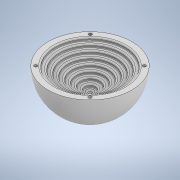
# Autodesk Inventor part: Energy_D
Saved by Autodesk Inventor 2022 (Build 260153000, 153)
## iProperties
Created: 2021-10-08
Part Number: Energy_D
Material: 一般
Document SubType Name: Modeling
Designer: zz091
Density: 1 g/cm^3
Appearance: 預設
Author: zz091
Autodesk Inventor part; units mm, degrees
ref_plane "YZ Plane" through (0, 0, 0) normal (1, 0, 0) x (0, 1, 0)
ref_plane "XZ Plane" through (0, 0, 0) normal (0, 1, 0) x (-1, 0, 0)
ref_plane "XY Plane" through (0, 0, 0) normal (0, 0, 1) x (1, 0, 0)
sketch "草圖3" plane through (0, 0, 0) normal (0, 1, 0) x (-1, 0, 0)
  circle A0 centre (0, 0) radius 30
  dimension "d1" = 60
  constraints: 1 centre point, 1 coincident
  measures "d1" diameter of A0
extrude "擠出1" add sketch "草圖3" against normal blind 30
fillet "圓角1" radius 30 1 edges at (30, -30, 0)
sketch "草圖4" plane through (0, 0, 0) normal (0, 1, 0) x (1, 0, 0)
  circle A0 centre (0, 0) radius 25
  dimension "d6" = 50
  constraints: 1 centre point, 1 coincident
  measures "d6" diameter of A0
extrude "擠出2" cut sketch "草圖4" against normal blind 2
sketch "草圖5" plane through (0, -2, 0) normal (0, 1, 0) x (1, 0, 0)
  circle A0 centre (0, 0) radius 22
  dimension "d9" = 44
  constraints: 1 centre point, 1 coincident
  measures "d9" diameter of A0
extrude "擠出3" cut sketch "草圖5" against normal blind 2
sketch "草圖6" plane through (0, -4, 0) normal (0, 1, 0) x (1, 0, 0)
  circle A0 centre (0, 0) radius 19
  dimension "d12" = 38
  constraints: 1 centre point, 1 coincident
  measures "d12" diameter of A0
extrude "擠出4" cut sketch "草圖6" against normal blind 2
sketch "草圖7" plane through (0, -6, 0) normal (0, 1, 0) x (1, 0, 0)
  circle A0 centre (0, 0) radius 16
  dimension "d15" = 32
  constraints: 1 centre point, 1 coincident
  measures "d15" diameter of A0
extrude "擠出5" cut sketch "草圖7" against normal blind 2
sketch "草圖8" plane through (0, -8, 0) normal (0, 1, 0) x (1, 0, 0)
  circle A0 centre (0, 0) radius 13
  dimension "d18" = 26
  constraints: 1 centre point, 1 coincident
  measures "d18" diameter of A0
extrude "擠出6" cut sketch "草圖8" against normal blind 2
sketch "草圖9" plane through (0, -10, 0) normal (0, 1, 0) x (1, 0, 0)
  circle A0 centre (0, 0) radius 10
  dimension "d21" = 20
  constraints: 1 centre point, 1 coincident
  measures "d21" diameter of A0
extrude "擠出7" cut sketch "草圖9" against normal blind 2
sketch "草圖10" plane through (0, -12, 0) normal (0, 1, 0) x (1, 0, 0)
  circle A0 centre (0, 0) radius 7
  dimension "d24" = 14
  constraints: 1 centre point, 1 coincident
  measures "d24" diameter of A0
extrude "擠出8" cut sketch "草圖10" against normal blind 2
sketch "草圖11" plane through (0, -14, 0) normal (0, 1, 0) x (1, 0, 0)
  circle A0 centre (0, 0) radius 4
  dimension "d27" = 8
  constraints: 1 centre point, 1 coincident
  measures "d27" diameter of A0
extrude "擠出9" cut sketch "草圖11" against normal blind 2
sketch "草圖14" plane through (0, -16, 0) normal (0, 1, 0) x (1, 0, 0)
  circle A0 centre (0, 0) radius 7 projected
  circle A1 centre (0, 0) radius 1.5
  dimension "d33" = 3
  constraints: 1 centre point, 1 coincident
  measures "d33" diameter of A1
extrude "擠出11" cut sketch "草圖14" against normal blind 2 contours A1
sketch "草圖15" plane through (0, 0, 0) normal (1, 0, 0) x (0, 1, 0)
  circle A0 centre (0, 0) radius 1.5
  dimension "d36" = 3
  constraints: 1 centre point, 1 coincident
  measures "d36" diameter of A0
extrude "擠出12" [suppressed]
sketch "草圖16" plane through (0, 0, 0) normal (0, 0, 1) x (1, 0, 0)
  circle A0 centre (0, 0) radius 1.5
  dimension "d41" = 3
  constraints: 1 centre point, 1 coincident
  measures "d41" diameter of A0
extrude "擠出13" [suppressed]
sketch "草圖25" plane through (0, 0, 0) normal (0, 0, 1) x (1, 0, 0)
  line L0 (0, 0) -> (24.7511, -24.7511)
  line L1 (30, 0) -> (30, 0) projected
  line L2 (0, 0) -> (25.9967, -23.4076)
  line L3 (24.7511, -24.7511) -> (25.9769, -23.3897)
  line L4 (0, 0) -> (23.4422, -26.0352)
  line L5 (23.4422, -26.0352) -> (24.7511, -24.7511)
  dimension "d63" = 45
  dimension "d64" = 3
  dimension "d69" = 42
  dimension "d70" = 48
  constraints: 10 end point, 1 perpendicular, 1 point on line
  measures "d63" angle of L1 L0
  measures "d64" angle of L2 L0
  measures "d69" angle of L1 L2
  measures "d70" angle of L1 L4
extrude "擠出16" [suppressed]
fillet "圓角2" [suppressed]
sketch "草圖26" plane through (0, 0, 0) normal (0, 0, 1) x (1, 0, 0)
  line L0 (0, 0) -> (-28.2843, -28.2843)
  line L1 (0, 0) -> (-29.7258, -26.7652)
  line L2 (0, 0) -> (-26.7652, -29.7258)
  line L3 (30, 0) -> (30, 0) projected
  line L4 (-26.7652, -29.7258) -> (-28.2455, -28.2455)
  line L5 (-28.2455, -28.2455) -> (-29.7258, -26.7652)
  dimension "d72" = 45
  dimension "d73" = 48
  dimension "d74" = 42
  dimension "d75" = 40
  dimension "d76" = 40
  dimension "d77" = 40
  constraints: 10 end point, 1 perpendicular, 1 point on line
  measures "d72" angle of L3 L0
  measures "d73" angle of L3 L2
  measures "d74" angle of L3 L1
  measures "d75" distance of L0.start L2.end
  measures "d76" distance of L0.start L0.end
  measures "d77" distance of L0.start L1.end
extrude "擠出17" [suppressed]
fillet "圓角3" [suppressed]
sketch "草圖27" plane through (0, 0, 0) normal (1, 0, 0) x (0, 1, 0)
  arc A0 (0, 0) -> (0, 0) centre (0, 0) ccw projected
  line L0 (0, 0) -> (-28.2843, 28.2843)
  line L1 (0, 0) -> (0, 0) projected
  line L2 (0, 0) -> (-26.9265, 29.9049)
  line L3 (0, 0) -> (-29.7666, 26.802)
  line L4 (-29.7666, 26.802) -> (-28.2843, 28.2843)
  line L5 (-28.2843, 28.2843) -> (-26.802, 29.7666)
  line L6 (0, 0) -> (-28.2843, -28.2843)
  line L7 (0, 0) -> (0, 0) projected
  line L8 (0, 0) -> (-26.8123, -29.7781)
  line L9 (0, 0) -> (-29.8282, -26.8575)
  line L10 (-28.2843, -28.2843) -> (-26.8123, -29.7781)
  line L11 (-28.2843, -28.2843) -> (-29.8282, -26.8575)
  point P0 (-1.1147, 1.0037)
  point P1 (-1.0607, 1.0607)
  point P2 (-1.0037, -1.1147)
  point P3 (-1.1147, -1.0037)
  point P4 (-1.0037, 1.1147)
  dimension "d83" = 40
  dimension "d84" = 45
  dimension "d85" = 42
  dimension "d86" = 48
  dimension "d87" = 45
  dimension "d88" = 40
  dimension "d89" = 42
  dimension "d90" = 48
  constraints: 20 end point, 2 point on line, 1 perpendicular, 1 other
  measures "d83" distance of L0.start L0.end
  measures "d84" angle of L1 L0
  measures "d85" angle of L1 L2
  measures "d86" angle of L1 L3
  measures "d87" angle of L7 L6
  measures "d88" distance of L0.start L6.end
  measures "d89" angle of L7 L8
  measures "d90" angle of L7 L9
extrude "擠出18" [suppressed]
fillet "圓角4" [suppressed]
sketch "草圖29" plane through (0, 0, 0) normal (0, 1, 0) x (1, 0, 0)
  circle A0 centre (-19.445, 19.6574) radius 1.15
  arc A1 (25, 0) -> (25, 0) centre (0, 0) ccw projected
  arc A2 (30, 0) -> (30, 0) centre (0, 0) ccw projected
  circle A3 centre (19.445, 19.4459) radius 1.15
  arc A4 (30, 0) -> (30, 0) centre (0, 0) ccw projected
  arc A5 (25, 0) -> (25, 0) centre (0, 0) ccw projected
  circle A6 centre (-19.445, -19.4459) radius 1.15
  arc A7 (25, 0) -> (25, 0) centre (0, 0) ccw projected
  circle A8 centre (19.445, -19.4459) radius 1.15
  dimension "d97" = 2.3
  dimension "d99" = 1.2
  dimension "d100" = 19.445
  dimension "d102" = 27.65
  dimension "d104" = 2.3
  dimension "d105" = 27.5
  dimension "d106" = 19.445
  dimension "d107" = 1.35
  dimension "d109" = 1.35
  dimension "d110" = 1.5
  dimension "d111" = 2.3
  dimension "d112" = 27.5
  dimension "d113" = 19.445
  dimension "d114" = 19.4459
  dimension "d117" = 2.3
  dimension "d118" = 27.5
  dimension "d119" = 19.445
  constraints: 4 centre point
  measures "d97" diameter of A0
  measures "d100" horizontal distance of point (0, 0) A0.centre
  measures "d102" distance of point (0, 0) A0.centre
  measures "d104" diameter of A3
  measures "d105" distance of A3.centre point (0, 0)
  measures "d106" horizontal distance of point (0, 0) A3.centre
  measures "d111" diameter of A6
  measures "d112" distance of A6.centre point (0, 0)
  measures "d113" horizontal distance of point (0, 0) A6.centre
  measures "d114" vertical distance of A6.centre point (0, 0)
  measures "d117" diameter of A8
  measures "d118" distance of point (0, 0) A8.centre
  measures "d119" horizontal distance of point (0, 0) A8.centre
extrude "擠出19" cut sketch "草圖29" against normal blind 3.5 contours A0 | A3 | A6 | A8
fillet "圓角5" radius 1 9 edges at (-25, 0, 0) (-22, -2, 0) (-19, -4, 0) (-16, -6, 0) (-13, -8, 0) (-10, -10, 0) (-7, -12, 0) (-4, -14, 0) (-1.5, -16, 0)
fillet "面圓角1" radius 0.382 1 edges at (-25, -2, 0)
fillet "面圓角2" radius 0.382 1 edges at (-22, -4, 0)
fillet "面圓角3" radius 0.382 1 edges at (-19, -6, 0)
fillet "面圓角4" radius 0.382 1 edges at (-16, -8, 0)
fillet "面圓角5" radius 0.382 1 edges at (-13, -10, 0)
fillet "面圓角6" radius 0.382 1 edges at (-10, -12, 0)
fillet "面圓角7" radius 0.382 1 edges at (-7, -14, 0)
fillet "面圓角8" radius 0.382 1 edges at (-4, -16, 0)
sketch "草圖30" plane through (0, -18, 0) normal (0, 1, 0) x (1, 0, 0)
  circle A0 centre (0, 0) radius 1.25
  dimension "d131" = 2.5
  constraints: 1 centre point, 1 coincident
  measures "d131" diameter of A0
extrude "擠出20" [suppressed]
feature "面圓角9" [suppressed]
fillet "圓角6" [suppressed]
